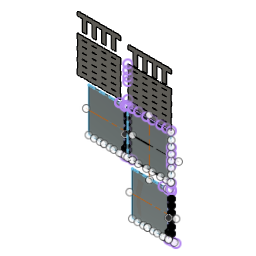
slowlab_solaroven_outside_box (Autodesk Fusion 360 design; units mm, degrees)
Autodesk Fusion 360 part; units mm, degrees
(part 1 of 2)
sketch "Sketch1" plane through (0, 0, 0) normal (0, 1, 0) x (1, 0, 0) in component "front"
  line L0 (0, 0) -> (300, 0)
  line L1 (300, 0) -> (300, -250)
  line L2 (300, -250) -> (0, -250)
  line L3 (0, -250) -> (0, 0)
  line L4 (33.1119, -2.5) -> (72.8619, -2.5)
  line L5 (72.8619, -2.5) -> (72.8619, 0)
  line L6 (72.8619, 0) -> (33.1119, 0)
  line L7 (33.1119, 0) -> (33.1119, -2.5)
  line L8 (227.1613, -2.5) -> (266.9113, -2.5)
  line L9 (266.9113, -2.5) -> (266.9113, 0)
  line L10 (266.9113, 0) -> (227.1613, 0)
  line L11 (227.1613, 0) -> (227.1613, -2.5)
  line L12 (130.0571, -2.5) -> (169.8071, -2.5)
  line L13 (169.8071, -2.5) -> (169.8071, 0)
  line L14 (169.8071, 0) -> (130.0571, 0)
  line L15 (130.0571, 0) -> (130.0571, -2.5)
  line L16 (0, -1.25) -> (33.0887, -1.25) construction
  line L17 (72.8915, -1.25) -> (130.1632, -1.25) construction
  line L18 (300, -212.3058) -> (297.5, -212.3058)
  line L19 (297.5, -212.3058) -> (297.5, -172.5558)
  line L20 (297.5, -172.5558) -> (300, -172.5558)
  line L21 (300, -172.5558) -> (300, -212.3058)
  line L22 (300, -144.875) -> (297.5, -144.875)
  line L23 (297.5, -144.875) -> (297.5, -105.125)
  line L24 (297.5, -105.125) -> (300, -105.125)
  line L25 (300, -105.125) -> (300, -144.875)
  line L26 (300, -77.4442) -> (297.5, -77.4442)
  line L27 (297.5, -77.4442) -> (297.5, -37.6942)
  line L28 (297.5, -37.6942) -> (300, -37.6942)
  line L29 (300, -37.6942) -> (300, -77.4442)
  line L30 (298.75, -250) -> (298.75, -212.3058) construction
  line L31 (298.75, -172.5558) -> (298.75, -144.875) construction
  line L32 (298.75, -105.125) -> (298.75, -77.4442) construction
  line L33 (298.75, -37.6942) -> (298.75, 0) construction
  line L34 (0, -37.6942) -> (2.5, -37.6942)
  line L35 (2.5, -37.6942) -> (2.5, -77.4442)
  line L36 (2.5, -77.4442) -> (0, -77.4442)
  line L37 (0, -77.4442) -> (0, -37.6942)
  line L38 (0, -105.125) -> (2.5, -105.125)
  line L39 (2.5, -105.125) -> (2.5, -144.875)
  line L40 (2.5, -144.875) -> (0, -144.875)
  line L41 (0, -144.875) -> (0, -105.125)
  line L42 (0, -172.5558) -> (2.5, -172.5558)
  line L43 (2.5, -172.5558) -> (2.5, -212.3058)
  line L44 (2.5, -212.3058) -> (0, -212.3058)
  line L45 (0, -212.3058) -> (0, -172.5558)
  line L46 (1.25, 0) -> (1.25, -37.6942) construction
  line L47 (1.25, -77.4442) -> (1.25, -105.125) construction
  line L48 (1.25, -144.875) -> (1.25, -172.5558) construction
  line L49 (1.25, -212.3058) -> (1.25, -250) construction
  line L50 (35.3369, -225.4541) -> (65.3369, -225.4541)
  line L51 (65.3369, -225.4541) -> (65.3369, -222.9541)
  line L52 (65.3369, -222.9541) -> (35.3369, -222.9541)
  line L53 (35.3369, -222.9541) -> (35.3369, -225.4541)
  line L54 (102.0036, -225.4541) -> (132.0036, -225.4541)
  line L55 (132.0036, -222.9541) -> (102.0036, -222.9541)
  line L56 (132.0036, -225.4541) -> (132.0036, -222.9541)
  line L57 (102.0036, -222.9541) -> (102.0036, -225.4541)
  line L58 (168.6703, -225.4541) -> (198.6703, -225.4541)
  line L59 (198.6703, -222.9541) -> (168.6703, -222.9541)
  line L60 (198.6703, -225.4541) -> (198.6703, -222.9541)
  line L61 (168.6703, -222.9541) -> (168.6703, -225.4541)
  line L62 (235.3369, -225.4541) -> (265.3369, -225.4541)
  line L63 (265.3369, -222.9541) -> (235.3369, -222.9541)
  line L64 (265.3369, -225.4541) -> (265.3369, -222.9541)
  line L65 (235.3369, -222.9541) -> (235.3369, -225.4541)
  line L66 (35.3369, -187.4541) -> (65.3369, -187.4541)
  line L67 (65.3369, -184.9541) -> (35.3369, -184.9541)
  line L68 (65.3369, -187.4541) -> (65.3369, -184.9541)
  line L69 (35.3369, -184.9541) -> (35.3369, -187.4541)
  line L70 (102.0036, -187.4541) -> (132.0036, -187.4541)
  line L71 (132.0036, -184.9541) -> (102.0036, -184.9541)
  line L72 (132.0036, -187.4541) -> (132.0036, -184.9541)
  line L73 (102.0036, -184.9541) -> (102.0036, -187.4541)
  line L74 (168.6703, -187.4541) -> (198.6703, -187.4541)
  line L75 (198.6703, -184.9541) -> (168.6703, -184.9541)
  line L76 (198.6703, -187.4541) -> (198.6703, -184.9541)
  line L77 (168.6703, -184.9541) -> (168.6703, -187.4541)
  line L78 (235.3369, -187.4541) -> (265.3369, -187.4541)
  line L79 (265.3369, -184.9541) -> (235.3369, -184.9541)
  line L80 (265.3369, -187.4541) -> (265.3369, -184.9541)
  line L81 (235.3369, -184.9541) -> (235.3369, -187.4541)
  line L82 (35.3369, -149.4541) -> (65.3369, -149.4541)
  line L83 (65.3369, -146.9541) -> (35.3369, -146.9541)
  line L84 (65.3369, -149.4541) -> (65.3369, -146.9541)
  line L85 (35.3369, -146.9541) -> (35.3369, -149.4541)
  line L86 (102.0036, -149.4541) -> (132.0036, -149.4541)
  line L87 (132.0036, -146.9541) -> (102.0036, -146.9541)
  line L88 (132.0036, -149.4541) -> (132.0036, -146.9541)
  line L89 (102.0036, -146.9541) -> (102.0036, -149.4541)
  line L90 (168.6703, -149.4541) -> (198.6703, -149.4541)
  line L91 (198.6703, -146.9541) -> (168.6703, -146.9541)
  line L92 (198.6703, -149.4541) -> (198.6703, -146.9541)
  line L93 (168.6703, -146.9541) -> (168.6703, -149.4541)
  line L94 (235.3369, -149.4541) -> (265.3369, -149.4541)
  line L95 (265.3369, -146.9541) -> (235.3369, -146.9541)
  line L96 (265.3369, -149.4541) -> (265.3369, -146.9541)
  line L97 (235.3369, -146.9541) -> (235.3369, -149.4541)
  line L98 (35.3369, -111.4541) -> (65.3369, -111.4541)
  line L99 (65.3369, -108.9541) -> (35.3369, -108.9541)
  line L100 (65.3369, -111.4541) -> (65.3369, -108.9541)
  line L101 (35.3369, -108.9541) -> (35.3369, -111.4541)
  line L102 (102.0036, -111.4541) -> (132.0036, -111.4541)
  line L103 (132.0036, -108.9541) -> (102.0036, -108.9541)
  line L104 (132.0036, -111.4541) -> (132.0036, -108.9541)
  line L105 (102.0036, -108.9541) -> (102.0036, -111.4541)
  line L106 (168.6703, -111.4541) -> (198.6703, -111.4541)
  line L107 (198.6703, -108.9541) -> (168.6703, -108.9541)
  line L108 (198.6703, -111.4541) -> (198.6703, -108.9541)
  line L109 (168.6703, -108.9541) -> (168.6703, -111.4541)
  line L110 (235.3369, -111.4541) -> (265.3369, -111.4541)
  line L111 (265.3369, -108.9541) -> (235.3369, -108.9541)
  line L112 (265.3369, -111.4541) -> (265.3369, -108.9541)
  line L113 (235.3369, -108.9541) -> (235.3369, -111.4541)
  line L114 (35.3369, -73.4541) -> (65.3369, -73.4541)
  line L115 (65.3369, -70.9541) -> (35.3369, -70.9541)
  line L116 (65.3369, -73.4541) -> (65.3369, -70.9541)
  line L117 (35.3369, -70.9541) -> (35.3369, -73.4541)
  line L118 (102.0036, -73.4541) -> (132.0036, -73.4541)
  line L119 (132.0036, -70.9541) -> (102.0036, -70.9541)
  line L120 (132.0036, -73.4541) -> (132.0036, -70.9541)
  line L121 (102.0036, -70.9541) -> (102.0036, -73.4541)
  line L122 (168.6703, -73.4541) -> (198.6703, -73.4541)
  line L123 (198.6703, -70.9541) -> (168.6703, -70.9541)
  line L124 (198.6703, -73.4541) -> (198.6703, -70.9541)
  line L125 (168.6703, -70.9541) -> (168.6703, -73.4541)
  line L126 (235.3369, -73.4541) -> (265.3369, -73.4541)
  line L127 (265.3369, -70.9541) -> (235.3369, -70.9541)
  line L128 (265.3369, -73.4541) -> (265.3369, -70.9541)
  line L129 (235.3369, -70.9541) -> (235.3369, -73.4541)
  line L130 (35.3369, -35.4541) -> (65.3369, -35.4541)
  line L131 (65.3369, -32.9541) -> (35.3369, -32.9541)
  line L132 (65.3369, -35.4541) -> (65.3369, -32.9541)
  line L133 (35.3369, -32.9541) -> (35.3369, -35.4541)
  line L134 (102.0036, -35.4541) -> (132.0036, -35.4541)
  line L135 (132.0036, -32.9541) -> (102.0036, -32.9541)
  line L136 (132.0036, -35.4541) -> (132.0036, -32.9541)
  line L137 (102.0036, -32.9541) -> (102.0036, -35.4541)
  line L138 (168.6703, -35.4541) -> (198.6703, -35.4541)
  line L139 (198.6703, -32.9541) -> (168.6703, -32.9541)
  line L140 (198.6703, -35.4541) -> (198.6703, -32.9541)
  line L141 (168.6703, -32.9541) -> (168.6703, -35.4541)
  line L142 (235.3369, -35.4541) -> (265.3369, -35.4541)
  line L143 (265.3369, -32.9541) -> (235.3369, -32.9541)
  line L144 (265.3369, -35.4541) -> (265.3369, -32.9541)
  line L145 (235.3369, -32.9541) -> (235.3369, -35.4541)
  line L146 (169.8896, -1.25) -> (227.1613, -1.25) construction
  line L147 (266.9113, -1.25) -> (300, -1.25) construction
  dimension "d3" = 300
  dimension "d4" = 250
  dimension "d14" = 39.75
  dimension "d15" = 39.75
  dimension "d17" = 39.75
  dimension "d18" = 39.75
  dimension "d19" = 2.5
  dimension "d20" = 39.75
  dimension "d21" = 2.5
  dimension "d22" = 39.75
  dimension "d23" = 2.5
  dimension "d24" = 39.75
  dimension "d25" = 39.75
  dimension "d26" = 39.75
  dimension "d27" = 2.5
  dimension "d28" = 2.5
  dimension "d85" = 30
  dimension "d86" = 2.5
  dimension "d89" = 200
  dimension "d90" = 190
  constraint horizontal L0
  constraint vertical L1
  constraint horizontal L2
  constraint vertical L3
  constraint coincident L0.start L3.end
  constraint horizontal L4
  constraint vertical L5
  constraint horizontal L6
  constraint vertical L7
  constraint coincident L0 L5.end
  constraint horizontal L8
  constraint vertical L9
  constraint horizontal L10
  constraint vertical L11
  constraint coincident L0 L9.end
  constraint horizontal L12
  constraint vertical L13
  constraint horizontal L14
  constraint vertical L15
  constraint coincident L0 L13.end
  constraint coincident L3 L16.start
  constraint perpendicular L3 L16
  constraint horizontal L18
  constraint vertical L19
  constraint horizontal L20
  constraint vertical L21
  constraint coincident L1 L18.start
  constraint horizontal L22
  constraint vertical L23
  constraint horizontal L24
  constraint vertical L25
  constraint coincident L1 L22.start
  constraint horizontal L26
  constraint vertical L27
  constraint horizontal L28
  constraint vertical L29
  constraint coincident L1 L26.start
  constraint coincident L2 L30.start
  constraint perpendicular L2 L30
  constraint midpoint L18 L30.end
  constraint midpoint L20 L31.start
  constraint midpoint L22 L31.end
  constraint midpoint L24 L32.start
  constraint midpoint L26 L32.end
  constraint midpoint L28 L33.start
  constraint coincident L0 L33.end
  constraint perpendicular L0 L33
  constraint equal L30 L33
  constraint equal L31 L32
  constraint horizontal L34
  constraint vertical L35
  constraint horizontal L36
  constraint vertical L37
  constraint coincident L3 L34.start
  constraint horizontal L38
  constraint vertical L39
  constraint horizontal L40
  constraint vertical L41
  constraint coincident L3 L38.start
  constraint horizontal L42
  constraint vertical L43
  constraint horizontal L44
  constraint vertical L45
  constraint coincident L3 L42.start
  constraint coincident L0 L46.start
  constraint perpendicular L0 L46
  constraint midpoint L34 L46.end
  constraint midpoint L36 L47.start
  constraint midpoint L38 L47.end
  constraint perpendicular L38 L47
  constraint midpoint L40 L48.start
  constraint midpoint L42 L48.end
  constraint midpoint L44 L49.start
  constraint coincident L2 L49.end
  constraint perpendicular L2 L49
  constraint equal L47 L48
  constraint equal L33 L46
  constraint equal L30 L49
  constraint horizontal L50
  constraint vertical L51
  constraint horizontal L52
  constraint vertical L53
  constraint midpoint L11 L146.end
  constraint midpoint L9 L147.start
  constraint coincident L1 L147.end
  constraint perpendicular L1 L147
  constraint equal L16 L147
  constraint equal L17 L146
  measures "d3" distance of L1.end L2.end
  measures "d4" distance of L0.start L2.end
  measures "d14" distance of L4.start L4.end
  measures "d15" distance of L12.start L12.end
  measures "d17" distance of L8.start L8.end
  measures "d18" distance of L18.end L19.end
  measures "d19" distance of L18.start L18.end
  measures "d20" distance of L22.end L23.end
  measures "d21" distance of L22.start L22.end
  measures "d22" distance of L26.end L27.end
  measures "d23" distance of L26.start L26.end
  measures "d24" distance of L34.end L35.end
  measures "d25" distance of L38.end L39.end
  measures "d26" distance of L42.end L43.end
  measures "d27" distance of L35.end L36.end
  measures "d28" distance of L42.start L42.end
  measures "d85" distance of L50.start L50.end
  measures "d86" distance of L50.end L51.end
extrude "Extrude1" add sketch "Sketch1" along normal blind 2.5 contours L0 L1 L2 L3 L4 L5 L7 L8 L9 L11 L12 L13 L15 L18 L19 L20 L22 L23 L24 L26 L27 L28 L34 L35 L36 L38 L39 L40 L42 L43 L44 makes body 1 in component "front"
sketch "Sketch1 (2)" plane through (0, 0, 0) normal (0, 1, 0) x (1, 0, 0) in component "side"
  line L0 (-18.915, 9.6817) -> (-268.915, 9.6817)
  line L1 (-268.915, 9.6817) -> (-268.915, 309.6817)
  line L2 (-268.915, 309.6817) -> (-18.915, 309.6817)
  line L3 (-18.915, 309.6817) -> (-18.915, 9.6817)
  line L4 (-18.915, 12.1817) -> (-56.6092, 12.1817)
  line L5 (-56.6092, 12.1817) -> (-56.6092, 9.6817)
  line L6 (-56.6092, 9.6817) -> (-18.915, 9.6817)
  line L7 (-18.915, 9.6817) -> (-18.915, 12.1817)
  line L8 (-231.2208, 9.6817) -> (-268.915, 9.6817)
  line L9 (-268.915, 9.6817) -> (-268.915, 12.1817)
  line L10 (-268.915, 12.1817) -> (-231.2208, 12.1817)
  line L11 (-231.2208, 12.1817) -> (-231.2208, 9.6817)
  line L12 (0, -250) -> (0, -212.3058)
  line L13 (-191.2208, 9.6817) -> (-163.54, 9.6817)
  line L14 (-163.54, 9.6817) -> (-163.54, 12.1817)
  line L15 (-163.54, 12.1817) -> (-191.2208, 12.1817)
  line L16 (-191.2208, 12.1817) -> (-191.2208, 9.6817)
  line L17 (0, -172.5558) -> (0, -144.875)
  line L18 (-231.2208, 10.9317) -> (-191.2208, 10.9317) construction
  line L19 (-123.54, 9.6817) -> (-96.6092, 9.6817)
  line L20 (-96.6092, 9.6817) -> (-96.6092, 12.1817)
  line L21 (-96.6092, 12.1817) -> (-123.54, 12.1817)
  line L22 (-123.54, 12.1817) -> (-123.54, 9.6817)
  line L23 (0, -37.6942) -> (0, 0)
  line L24 (-96.6092, 10.9317) -> (-56.6092, 10.9317) construction
  line L25 (-163.54, 10.9317) -> (-123.54, 10.9317) construction
  line L26 (-286.6858, 159.6817) -> (32.558, 159.6817)
  line L27 (-268.915, 307.1817) -> (-231.2208, 307.1817)
  line L28 (-268.915, 309.6817) -> (-268.915, 307.1817)
  line L29 (-231.2208, 307.1817) -> (-231.2208, 309.6817)
  line L30 (-191.2208, 307.1817) -> (-191.2208, 309.6817)
  line L31 (-163.54, 307.1817) -> (-191.2208, 307.1817)
  line L32 (-163.54, 309.6817) -> (-163.54, 307.1817)
  line L33 (-123.54, 307.1817) -> (-123.54, 309.6817)
  line L34 (-96.6092, 307.1817) -> (-123.54, 307.1817)
  line L35 (-96.6092, 309.6817) -> (-96.6092, 307.1817)
  line L36 (-56.6092, 307.1817) -> (-56.6092, 309.6817)
  line L37 (-18.915, 307.1817) -> (-56.6092, 307.1817)
  line L38 (-18.915, 309.6817) -> (-18.915, 307.1817)
  point P0 (-163.54, 308.4317)
  dimension "d31" = 250
  dimension "d32" = 300
  dimension "d33" = 2.5
  dimension "d36" = 2.5
  dimension "d37" = 40
  dimension "d38" = 2.5
  dimension "d39" = 2.5
  dimension "d40" = 40
  dimension "d41" = 40
  constraint horizontal L0
  constraint vertical L1
  constraint horizontal L2
  constraint vertical L3
  constraint horizontal L4
  constraint vertical L5
  constraint horizontal L6
  constraint vertical L7
  constraint coincident L0 L5.end
  constraint coincident L3 L4.start
  constraint horizontal L8
  constraint vertical L9
  constraint horizontal L10
  constraint vertical L11
  constraint coincident L1 L9.end
  constraint coincident L0 L8.start
  constraint equal L10 L12
  constraint horizontal L13
  constraint vertical L14
  constraint horizontal L15
  constraint vertical L16
  constraint coincident L0 L13.start
  constraint equal L15 L17
  constraint midpoint L11 L18.start
  constraint midpoint L16 L18.end
  constraint horizontal L19
  constraint vertical L20
  constraint horizontal L21
  constraint vertical L22
  constraint coincident L0 L19.start
  constraint equal L4 L23
  constraint midpoint L20 L24.start
  constraint midpoint L5 L24.end
  constraint midpoint L14 L25.start
  constraint midpoint L22 L25.end
  constraint perpendicular L3 L26
  constraint symmetric L0 L2 L26
  constraint symmetric L4.start L26 L37.start
  constraint symmetric L4.end L26 L36.start
  constraint symmetric L5.end L26 L36.end
  constraint symmetric L0.start L26 L2.end
  constraint symmetric L8.start L26 L29.end
  constraint symmetric L0.end L26 L1.end
  constraint symmetric L9.end L26 L27.start
  constraint symmetric L10.end L26 L27.end
  constraint symmetric L13.start L26 L30.end
  constraint symmetric L13.end L26 L32.start
  constraint symmetric L14.end L26 L31.start
  constraint symmetric L15.end L26 L30.start
  constraint symmetric L19.start L26 L33.end
  constraint symmetric L19.end L26 L35.start
  constraint symmetric L20.end L26 L34.start
  constraint symmetric L21.end L26 L33.start
  constraint symmetric L25.start L26 P0
  measures "d31" distance of L0.start L0.end
  measures "d32" distance of L0.start L2.end
  measures "d33" distance of L8.start L10.end
  measures "d36" distance of L13.start L15.end
  measures "d37" distance of L18.start L18.end
  measures "d38" distance of L19.start L21.end
  measures "d39" distance of L4.end L5.end
  measures "d40" distance of L24.start L24.end
  measures "d41" distance of L25.start L25.end
sketch "Sketch1 (3)" plane through (0, 0, 0) normal (0, 1, 0) x (1, 0, 0) in component "base"
  line L0 (-1.0292, 9.6817) -> (298.9708, 9.6817)
  line L1 (298.9708, 9.6817) -> (298.9708, 309.6817)
  line L2 (298.9708, 309.6817) -> (-1.0292, 309.6817)
  line L3 (-1.0292, 309.6817) -> (-1.0292, 9.6817)
  line L4 (265.8821, 9.6817) -> (298.9708, 9.6817)
  line L5 (298.9708, 9.6817) -> (298.9708, 12.1817)
  line L6 (298.9708, 12.1817) -> (265.8821, 12.1817)
  line L7 (265.8821, 12.1817) -> (265.8821, 9.6817)
  line L8 (225.8821, 9.6817) -> (168.5279, 9.6817)
  line L9 (168.5279, 9.6817) -> (168.5279, 12.1817)
  line L10 (168.5279, 12.1817) -> (225.8821, 12.1817)
  line L11 (225.8821, 12.1817) -> (225.8821, 9.6817)
  line L12 (265.8821, 10.9317) -> (225.8821, 10.9317) construction
  line L13 (300, 0) -> (266.9113, 0)
  line L14 (227.1613, 0) -> (169.8071, 0)
  line L15 (129.2779, 9.6817) -> (72.0827, 9.6817)
  line L16 (72.0827, 9.6817) -> (72.0827, 12.1817)
  line L17 (72.0827, 12.1817) -> (129.2779, 12.1817)
  line L18 (129.2779, 12.1817) -> (129.2779, 9.6817)
  line L19 (32.0827, 9.6817) -> (-1.0292, 9.6817)
  line L20 (-1.0292, 9.6817) -> (-1.0292, 12.1817)
  line L21 (-1.0292, 12.1817) -> (32.0827, 12.1817)
  line L22 (32.0827, 12.1817) -> (32.0827, 9.6817)
  line L23 (33.1119, 0) -> (0, 0)
  line L24 (32.0827, 10.9317) -> (72.0827, 10.9317) construction
  line L25 (130.0571, 0) -> (72.8619, 0)
  line L26 (349.5665, 159.6817) -> (-8.1069, 159.6817) construction
  line L27 (-8.1069, 159.6817) -> (142.7167, 159.6817)
  line L28 (298.9708, 307.1817) -> (265.8821, 307.1817)
  line L29 (265.8821, 307.1817) -> (265.8821, 309.6817)
  line L30 (168.5279, 307.1817) -> (225.8821, 307.1817)
  line L31 (225.8821, 307.1817) -> (225.8821, 309.6817)
  line L32 (168.5279, 309.6817) -> (168.5279, 307.1817)
  line L33 (129.2779, 307.1817) -> (129.2779, 309.6817)
  line L34 (72.0827, 307.1817) -> (129.2779, 307.1817)
  line L35 (72.0827, 309.6817) -> (72.0827, 307.1817)
  line L36 (32.0827, 307.1817) -> (32.0827, 309.6817)
  line L37 (-1.0292, 307.1817) -> (32.0827, 307.1817)
  line L38 (-1.0292, 309.6817) -> (-1.0292, 307.1817)
  line L39 (-1.0292, 9.6817) -> (1.4708, 9.6817)
  line L40 (1.4708, 9.6817) -> (1.4708, 56.207)
  line L41 (1.4708, 56.207) -> (-1.0292, 56.207)
  line L42 (-1.0292, 56.207) -> (-1.0292, 9.6817)
  line L43 (-1.0292, 96.207) -> (1.4708, 96.207)
  line L44 (1.4708, 96.207) -> (1.4708, 139.6817)
  line L45 (1.4708, 139.6817) -> (-1.0292, 139.6817)
  line L46 (-1.0292, 139.6817) -> (-1.0292, 96.207)
  line L47 (0.2208, 56.207) -> (0.2208, 96.207) construction
  line L48 (-1.0292, 263.1564) -> (1.4708, 263.1564)
  line L49 (1.4708, 263.1564) -> (1.4708, 309.6817)
  line L50 (1.4708, 309.6817) -> (-1.0292, 309.6817)
  line L51 (-1.0292, 309.6817) -> (-1.0292, 263.1564)
  line L52 (-1.0292, 179.6817) -> (1.4708, 179.6817)
  line L53 (1.4708, 179.6817) -> (1.4708, 223.1564)
  line L54 (1.4708, 223.1564) -> (-1.0292, 223.1564)
  line L55 (-1.0292, 223.1564) -> (-1.0292, 179.6817)
  line L56 (0.2208, 139.6817) -> (0.2208, 179.6817) construction
  line L57 (0.2208, 223.1564) -> (0.2208, 263.1564) construction
  line L58 (148.9708, 369.1425) -> (148.9708, -19.3524) construction
  line L59 (296.4708, 9.6817) -> (296.4708, 56.207)
  line L60 (296.4708, 56.207) -> (298.9708, 56.207)
  line L61 (298.9708, 96.207) -> (296.4708, 96.207)
  line L62 (296.4708, 96.207) -> (296.4708, 139.6817)
  line L63 (296.4708, 139.6817) -> (298.9708, 139.6817)
  line L64 (296.4708, 179.6817) -> (296.4708, 223.1564)
  line L65 (298.9708, 179.6817) -> (296.4708, 179.6817)
  line L66 (296.4708, 223.1564) -> (298.9708, 223.1564)
  line L67 (298.9708, 263.1564) -> (296.4708, 263.1564)
  line L68 (296.4708, 263.1564) -> (296.4708, 309.6817)
  line L69 (-56.6092, 9.6817) -> (-18.915, 9.6817)
  point P0 (32.0827, 308.4317)
  dimension "d45" = 300
  dimension "d46" = 300
  dimension "d47" = 2.5
  dimension "d48" = 2.5
  dimension "d49" = 40
  dimension "d50" = 2.5
  dimension "d51" = 2.5
  dimension "d52" = 40
  dimension "d54" = 2.5
  dimension "d55" = 2.5
  dimension "d56" = 40
  dimension "d58" = 2.5
  dimension "d60" = 2.5
  dimension "d61" = 40
  dimension "d62" = 40
  constraint horizontal L0
  constraint vertical L1
  constraint horizontal L2
  constraint vertical L3
  constraint horizontal L4
  constraint vertical L5
  constraint horizontal L6
  constraint vertical L7
  constraint coincident L1 L5.end
  constraint coincident L0 L4.start
  constraint horizontal L8
  constraint vertical L9
  constraint horizontal L10
  constraint vertical L11
  constraint coincident L0 L8.start
  constraint midpoint L7 L12.start
  constraint midpoint L11 L12.end
  constraint equal L6 L13
  constraint equal L10 L14
  constraint horizontal L15
  constraint vertical L16
  constraint horizontal L17
  constraint vertical L18
  constraint coincident L0 L15.start
  constraint horizontal L19
  constraint vertical L20
  constraint horizontal L21
  constraint vertical L22
  constraint coincident L3 L20.end
  constraint coincident L0 L19.start
  constraint equal L21 L23
  constraint midpoint L22 L24.start
  constraint midpoint L16 L24.end
  constraint equal L17 L25
  constraint perpendicular L3 L26
  constraint coincident L26 L27.end
  constraint symmetric L0 L2 L26
  constraint symmetric L4.start L26 L29.end
  constraint symmetric L5.end L26 L28.start
  constraint symmetric L6.end L26 L28.end
  constraint symmetric L8.start L26 L31.end
  constraint symmetric L8.end L26 L32.start
  constraint symmetric L9.end L26 L30.start
  constraint symmetric L10.end L26 L30.end
  constraint symmetric L15.start L26 L33.end
  constraint symmetric L15.end L26 L35.start
  constraint symmetric L16.end L26 L34.start
  constraint symmetric L17.end L26 L33.start
  constraint symmetric L19.start L26 L36.end
  constraint symmetric L0.start L26 L2.end
  constraint symmetric L20.end L26 L37.start
  constraint symmetric L21.end L26 L36.start
  constraint symmetric L24.start L26 P0
  constraint horizontal L39
  constraint vertical L40
  constraint horizontal L41
  constraint vertical L42
  constraint horizontal L43
  constraint vertical L44
  constraint horizontal L45
  constraint vertical L46
  constraint coincident L3 L43.start
  constraint midpoint L41 L47.start
  constraint midpoint L43 L47.end
  constraint horizontal L48
  constraint vertical L49
  constraint horizontal L50
  constraint vertical L51
  constraint coincident L2 L49.end
  constraint coincident L3 L48.start
  constraint horizontal L52
  constraint vertical L53
  constraint horizontal L54
  constraint vertical L55
  constraint coincident L3 L52.start
  constraint midpoint L45 L56.start
  constraint midpoint L52 L56.end
  constraint midpoint L54 L57.start
  constraint midpoint L48 L57.end
  constraint equal L40 L49
  constraint equal L44 L53
  constraint perpendicular L0 L58
  constraint symmetric L39.end L58 L59.start
  constraint symmetric L40.end L58 L59.end
  constraint symmetric L41.end L58 L60.end
  constraint symmetric L43.start L58 L61.start
  constraint symmetric L43.end L58 L61.end
  constraint symmetric L44.end L58 L62.end
  constraint symmetric L45.end L58 L63.end
  constraint symmetric L48.start L58 L67.start
  constraint symmetric L48.end L58 L67.end
  constraint symmetric L49.end L58 L68.end
  constraint symmetric L52.start L58 L65.start
  constraint symmetric L52.end L58 L64.start
  constraint symmetric L53.end L58 L64.end
  constraint symmetric L54.end L58 L66.end
  constraint collinear L0 L69
  measures "d45" distance of L0.start L0.end
  measures "d46" distance of L0.start L2.end
  measures "d47" distance of L4.start L6.end
  measures "d48" distance of L8.start L10.end
  measures "d49" distance of L12.start L12.end
  measures "d50" distance of L19.start L21.end
  measures "d51" distance of L15.end L16.end
  measures "d52" distance of L24.start L24.end
  measures "d54" distance of L40.end L41.end
  measures "d55" distance of L43.start L43.end
  measures "d56" distance of L47.start L47.end
  measures "d58" distance of L48.start L48.end
  measures "d60" distance of L52.start L52.end
  measures "d61" distance of L56.start L56.end
  measures "d62" distance of L57.start L57.end
extrude "Extrude1'" add sketch "Sketch1 (3)" along normal blind 2.5 separate body contours L0 L1 L2 L3 L6 L7 L9 L10 L11 L16 L17 L18 L21 L22 L28 L29 L30 L31 L32 L33 L34 L35 L36 L37 L40 L41 L43 L44 L45 L48 L49 L52 L53 L54 L59 L60 L61 L62 L63 L64 L65 L66 L67 L68 makes body 2 in component "base"
sketch "Sketch2" plane through (0, 0, 0) normal (0, 1, 0) x (-1, 0, 0) in component "side"
  line L0 (21.415, -56.332) -> (18.915, -56.332)
  line L1 (18.915, -56.332) -> (18.915, -96.082)
  line L2 (18.915, -96.082) -> (21.415, -96.082)
  line L3 (21.415, -96.082) -> (21.415, -56.332)
  line L4 (18.915, -309.6817) -> (18.915, -9.6817)
  line L5 (28.2467, -9.6817) -> (15.3841, -9.6817) construction
  line L6 (56.6092, -9.6817) -> (18.915, -9.6817)
  line L7 (-1.4708, -56.207) -> (-1.4708, -12.1817)
  line L8 (21.415, -139.6638) -> (18.915, -139.6638)
  line L9 (18.915, -139.6638) -> (18.915, -179.4138)
  line L10 (18.915, -179.4138) -> (21.415, -179.4138)
  line L11 (21.415, -179.4138) -> (21.415, -139.6638)
  line L12 (-1.4708, -139.6817) -> (-1.4708, -96.207)
  line L13 (21.415, -223.2814) -> (18.915, -223.2814)
  line L14 (18.915, -223.2814) -> (18.915, -263.0314)
  line L15 (18.915, -263.0314) -> (21.415, -263.0314)
  line L16 (21.415, -263.0314) -> (21.415, -223.2814)
  line L17 (-1.4708, -223.1564) -> (-1.4708, -179.6817)
  line L18 (43.0756, -307.1817) -> (-19.8282, -307.1817) construction
  line L19 (-1.4708, -307.1817) -> (-32.0827, -307.1817)
  line L20 (20.165, -263.0314) -> (20.165, -304.2317) construction
  line L21 (-1.4708, -56.207) -> (-1.4708, -96.207) construction
  line L22 (-1.4708, -76.207) -> (21.415, -76.207) construction
  line L23 (-1.4708, -223.1564) -> (-1.4708, -263.1564) construction
  line L24 (-1.4708, -243.1564) -> (21.415, -243.1564) construction
  line L25 (-1.4708, -139.6817) -> (-1.4708, -179.6817) construction
  line L26 (-1.4708, -159.6817) -> (21.415, -159.6817) construction
  point P0 (-1.4708, -263.1564)
  dimension "d66" = 39.75
  dimension "d67" = 2.5
  dimension "d69" = 39.75
  dimension "d70" = 2.5
  dimension "d71" = 2.5
  dimension "d72" = 39.75
  constraint horizontal L0
  constraint vertical L1
  constraint horizontal L2
  constraint vertical L3
  constraint collinear L1 L4
  constraint perpendicular L4 L5
  constraint collinear L5 L6
  constraint horizontal L8
  constraint vertical L9
  constraint horizontal L10
  constraint vertical L11
  constraint coincident L4 L9.end
  constraint horizontal L13
  constraint vertical L14
  constraint horizontal L15
  constraint vertical L16
  constraint coincident L4 L14.end
  constraint horizontal L18
  constraint collinear L18 L19
  constraint midpoint L15 L20.start
  constraint perpendicular L18 L20
  constraint coincident L7.start L21.start
  constraint coincident L12.end L21.end
  constraint midpoint L21 L22.start
  constraint midpoint L3 L22.end
  constraint horizontal L22
  constraint coincident L17.start L23.start
  constraint coincident P0 L23.end
  constraint midpoint L23 L24.start
  constraint midpoint L16 L24.end
  constraint coincident L12.start L25.start
  constraint coincident L17.end L25.end
  constraint midpoint L25 L26.start
  constraint coincident L11 L26.end
  constraint parallel L24 L26
  constraint horizontal L26
  measures "d66" distance of L0.start L2.end
  measures "d67" distance of L1.end L2.end
  measures "d69" distance of L8.start L10.end
  measures "d70" distance of L9.end L10.end
  measures "d71" distance of L13.start L13.end
  measures "d72" distance of L13.start L15.end
extrude "Extrude5" add sketch "Sketch1 (2)" along normal blind 2.5 separate body contours L0 L1 L3 L4 L5 L10 L11 L14 L15 L16 L20 L21 L22 L26 | L1 L2 L3 L26 L27 L29 L30 L31 L32 L33 L34 L35 L36 L37 makes body 3 in component "side"
extrude "Extrude6" cut sketch "Sketch2" along normal through all bodies 3 in component "side"
sketch "Sketch1 (4)" plane through (0, 0, 0) normal (0, 1, 0) x (1, 0, 0) in component "ruler"
  line L0 (10, -367.5617) -> (290, -367.5617)
  line L1 (300, -357.5617) -> (300, -257.5617)
  line L2 (0, -257.5617) -> (0, -357.5617)
  line L3 (0, -300.6724) -> (0, -219.9539) construction
  line L4 (0, -250) -> (0, -212.3058)
  arc A0 (0, -357.5617) -> (10, -367.5617) centre (10, -357.5617) ccw
  arc A1 (290, -367.5617) -> (300, -357.5617) centre (290, -357.5617) ccw
  line L5 (35.3369, -215.4773) -> (35.3369, -343.9941) construction
  line L6 (35.3369, -225.4541) -> (35.3369, -222.9541)
  line L7 (0, -337.5617) -> (35.3369, -337.5617)
  line L8 (35.3369, -337.5617) -> (35.3369, -257.5617)
  line L9 (35.3369, -257.5617) -> (0, -257.5617)
  line L10 (0, -257.5617) -> (0, -337.5617)
  line L11 (168.6703, -307.5826) -> (168.6703, -220.9735) construction
  line L12 (235.3369, -307.5826) -> (235.3369, -216.7371) construction
  line L13 (102.0036, -297.5971) -> (102.0036, -220.9735) construction
  line L14 (102.0036, -225.4541) -> (102.0036, -222.9541)
  line L15 (168.6703, -225.4541) -> (168.6703, -222.9541)
  line L16 (235.3369, -225.4541) -> (235.3369, -222.9541)
  line L17 (132.0036, -337.5617) -> (168.6703, -337.5617)
  line L18 (168.6703, -337.5617) -> (168.6703, -257.5617)
  line L19 (168.6703, -257.5617) -> (132.0036, -257.5617)
  line L20 (132.0036, -257.5617) -> (132.0036, -337.5617)
  line L21 (198.6703, -337.5617) -> (235.3369, -337.5617)
  line L22 (235.3369, -337.5617) -> (235.3369, -257.5617)
  line L23 (235.3369, -257.5617) -> (198.6703, -257.5617)
  line L24 (198.6703, -257.5617) -> (198.6703, -337.5617)
  line L25 (265.3369, -337.5617) -> (300, -337.5617)
  line L26 (300, -337.5617) -> (300, -257.5617)
  line L27 (300, -257.5617) -> (265.3369, -257.5617)
  line L28 (265.3369, -257.5617) -> (265.3369, -337.5617)
  line L29 (0, -257.5617) -> (300, -257.5617)
  line L30 (-27.4532, -337.5617) -> (336.2685, -337.5617) construction
  line L31 (65.3369, -337.5617) -> (102.0036, -337.5617)
  line L32 (102.0036, -337.5617) -> (102.0036, -257.5617)
  line L33 (102.0036, -257.5617) -> (65.3369, -257.5617)
  line L34 (65.3369, -257.5617) -> (65.3369, -337.5617)
  point P0 (0, -367.5617)
  point P1 (300, -367.5617)
  dimension "d91" = 300
  dimension "d92" = 10
  dimension "d93" = 10
  dimension "d98" = 30
  dimension "d99" = 30
  dimension "d100" = 30
  dimension "d101" = 30
  constraint horizontal L0
  constraint vertical L1
  constraint vertical L2
  constraint collinear L3 L4
  constraint collinear L2 L3
  constraint coincident P0 L0
  constraint coincident P0 L2
  constraint tangent L0 A0
  constraint tangent L2 A0
  constraint coincident P1 L0
  constraint coincident P1 L1
  constraint tangent L0 A1
  constraint tangent L1 A1
  constraint collinear L5 L6
  constraint horizontal L7
  constraint vertical L8
  constraint horizontal L9
  constraint vertical L10
  constraint coincident L5 L8.end
  constraint coincident L2 L7.start
  constraint collinear L13 L14
  constraint collinear L11 L15
  constraint collinear L12 L16
  constraint horizontal L17
  constraint vertical L18
  constraint horizontal L19
  constraint vertical L20
  constraint horizontal L21
  constraint vertical L22
  constraint horizontal L23
  constraint vertical L24
  constraint collinear L11 L18
  constraint collinear L12 L22
  constraint horizontal L25
  constraint vertical L26
  constraint horizontal L27
  constraint vertical L28
  constraint perpendicular L1 L29
  constraint perpendicular L24 L30
  constraint horizontal L31
  constraint vertical L32
  constraint horizontal L33
  constraint vertical L34
  constraint coincident L13 L32.end
  constraint coincident L29 L32.end
  constraint coincident L30 L31.start
  measures "d91" distance of P0 P1
  measures "d92" radius of A0
  measures "d93" radius of A1
  measures "d98" distance of L18 L24
  measures "d99" distance of L22 L28
  measures "d100" distance of L20 L32
  measures "d101" distance of L5 L34
extrude "Extrude1''" add sketch "Sketch1 (4)" along normal blind 2.5 separate body contours L0 L1 L2 A0 A1 L7 L8 L17 L18 L20 L21 L22 L24 L25 L28 L29 L31 L32 L34 makes body 4 in component "ruler"